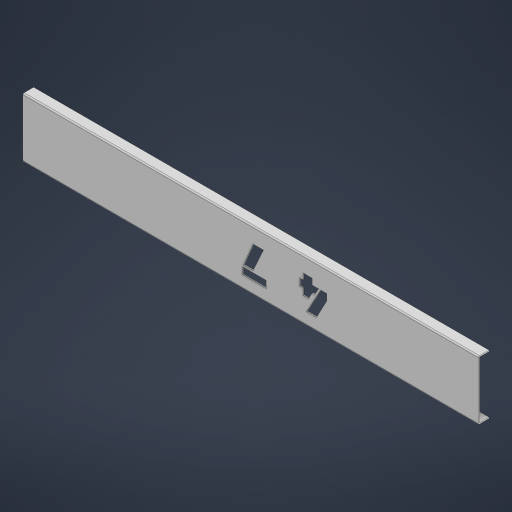
# Autodesk Inventor part: Chassis FrontandBack
Saved by Autodesk Inventor 2023 (Build 270158000, 158)
## iProperties
Created: 2022-04-13
Part Number: Chassis FrontandBack
Material: Generic
Document SubType Name: Modeling
Designer: timmy
Density: 1 g/cm^3
Appearance: Default
Author: timmy
Autodesk Inventor part; units mm, degrees
ref_plane "YZ Plane" through (0, 0, 0) normal (1, 0, 0) x (0, 1, 0)
ref_plane "XZ Plane" through (0, 0, 0) normal (0, 1, 0) x (-1, 0, 0)
ref_plane "XY Plane" through (0, 0, 0) normal (0, 0, 1) x (1, 0, 0)
sketch "Sketch1" plane through (0, 0, 0) normal (0, 0, 1) x (1, 0, 0)
  line L0 (0, 0) -> (609.6, 0)
  line L1 (609.6, 0) -> (609.6, 76.2)
  line L2 (609.6, 76.2) -> (0, 76.2)
  line L3 (0, 76.2) -> (0, 0)
  dimension "d0" = 609.6
  dimension "d1" = 76.2
  constraints: 8 end point, 2 parallel, 1 horizontal, 1 perpendicular
  measures "d0" distance of L2.end L1.end
  measures "d1" distance of L1.end L0.end
extrude "Extrusion1" add sketch "Sketch1" along normal blind 1.5875
sketch "Sketch2" plane through (0, 76.2, 0) normal (0, 1, 0) x (1, 0, 0)
  line L0 (609.6, 0) -> (0, 0) projected
  line L1 (0, 0) -> (0, -1.5875) projected
  line L2 (609.6, -1.5875) -> (0, -1.5875) projected
  line L3 (609.6, 0) -> (609.6, -1.5875) projected
  line L4 (609.6, -1.5875) -> (0, -1.5875)
  line L5 (0, -1.5875) -> (0, 12.7)
  line L6 (0, 12.7) -> (609.6, 12.7)
  line L7 (609.6, 12.7) -> (609.6, -1.5875)
  dimension "d39" = 12.7
  constraints: 8 end point, 2 parallel, 1 horizontal, 1 perpendicular
  measures "d39" distance between parallel lines of L6 L0
extrude "Extrusion2" add sketch "Sketch2" along normal blind 1.5875
fillet "Fillet1" radius 1.5875 1 edges at (304.8, 77.7875, 1.5875)
sketch "Sketch3" plane through (0, 0, 0) normal (0, -1, 0) x (1, 0, 0)
  line L0 (609.6, 0) -> (0, 0) projected
  line L1 (0, -12.7) -> (0, 0) projected
  line L2 (609.6, -12.7) -> (0, -12.7) projected
  line L3 (609.6, 0) -> (609.6, -12.7) projected
extrude "Extrusion3" add sketch "Sketch3" along normal blind 1.5875
sketch "Sketch4" plane through (0, 76.2, -12.7) normal (-1, 0, 0) x (0, 0, 1)
  line L0 (12.7, -76.2) -> (0, -76.2) projected
  line L1 (0, -76.2) -> (0, -77.7875) projected
  line L2 (12.7, -77.7875) -> (0, -77.7875) projected
  line L3 (12.7, -76.2) -> (12.7, -77.7875) projected
  arc A0 (14.2875, 0) -> (12.7, 1.5875) centre (12.7, 0) ccw projected
  line L4 (0, 1.5875) -> (12.7, 1.5875) projected
  line L5 (0, 0) -> (0, 1.5875) projected
  line L6 (0, 0) -> (12.7, 0) projected
  line L7 (12.7, 0) -> (12.7, -76.2) projected
  line L8 (12.7, -76.2) -> (14.2875, -76.2) projected
  line L9 (14.2875, -76.2) -> (14.2875, 0) projected
  line L10 (12.7, -76.2) -> (14.2875, -76.2)
  line L11 (14.2875, -76.2) -> (14.2875, -77.7875)
  line L12 (14.2875, -77.7875) -> (12.7, -77.7875)
  line L13 (12.7, -77.7875) -> (12.7, -76.2)
  constraints: 8 end point, 2 parallel, 1 horizontal, 1 perpendicular
extrude "Extrusion4" add sketch "Sketch4" against normal up to surface (609.6 mm away) contours L8 L11 L12 L3
fillet "Fillet2" radius 1.5875 1 edges at (304.8, -1.5875, 1.5875)
sketch "Sketch5" plane through (0, 0, 1.5875) normal (0, 0, 1) x (1, 0, 0)
  line L0 (391.8077, 9.2075) -> (217.7923, 9.2075) construction
  line L1 (217.7923, 9.2075) -> (217.7923, 67.0009) construction
  line L2 (217.7923, 67.0009) -> (391.8077, 67.0009) construction
  line L3 (391.8077, 67.0009) -> (391.8077, 9.2075) construction
  line L4 (392.9131, 14.4793) -> (379.4788, 14.4793)
  line L5 (379.4788, 14.4793) -> (398.5016, 49.12)
  line L6 (398.5016, 49.12) -> (406.8657, 49.12)
  line L7 (406.8657, 49.12) -> (406.8657, 40.7559)
  line L8 (406.8657, 40.7559) -> (392.9131, 14.4793)
  line L9 (390.2115, 39.5716) -> (386.9546, 39.5716)
  line L10 (386.9546, 39.5716) -> (382.3899, 30.9748)
  line L11 (382.3899, 30.9748) -> (374.9266, 30.9748)
  line L12 (374.9266, 30.9748) -> (374.9266, 39.5716)
  line L13 (374.9266, 39.5716) -> (369.7453, 39.5716)
  line L14 (369.7453, 39.5716) -> (369.7453, 49.12)
  line L15 (369.7453, 49.12) -> (374.9266, 49.12)
  line L16 (374.9266, 49.12) -> (374.9266, 57.1881)
  line L17 (374.9266, 57.1881) -> (386.9546, 57.1881)
  line L18 (386.9546, 57.1881) -> (386.9546, 49.12)
  line L19 (386.9546, 49.12) -> (395.8369, 49.12)
  line L20 (395.8369, 49.12) -> (390.2115, 39.5716)
  line L21 (308.0211, 26.3513) -> (322.0801, 57.1881)
  line L22 (322.0801, 57.1881) -> (308.0211, 57.1881)
  line L23 (308.0211, 57.1881) -> (295.1504, 26.3513)
  line L24 (295.1504, 26.3513) -> (308.0211, 26.3513)
  line L25 (325.5793, 14.4793) -> (325.5793, 23.894)
  line L26 (325.5793, 23.894) -> (293.6633, 23.894)
  line L27 (325.5793, 14.4793) -> (293.6633, 14.4793)
  line L28 (293.6633, 14.4793) -> (293.6633, 23.894)
  line L29 (352.5859, 14.2935) -> (352.5859, 45.4091)
  line L30 (350.864, 47.7439) -> (345.5928, 47.7439)
  line L31 (345.5928, 47.7439) -> (345.5928, 57.5211)
  line L32 (365.0153, 45.4091) -> (365.0153, 26.3513)
  arc A0 (352.5859, 45.4091) -> (350.901, 47.695) centre (350.286, 45.4778) ccw
  arc A1 (352.5859, 14.2935) -> (365.0153, 26.3513) centre (353.0272, 26.2737) ccw
  arc A2 (343.0715, 27.1984) -> (347.3973, 23.4081) centre (346.8949, 27.1984) ccw
  line L33 (343.0715, 57.5844) -> (343.0715, 27.1984)
  line L34 (349.8722, 23.894) -> (349.8722, 14.2935)
  line L35 (349.8722, 14.2935) -> (343.6768, 14.2935)
  arc A3 (330.9215, 25.1088) -> (343.6768, 14.2935) centre (342.4037, 25.7213) ccw
  line L36 (330.9215, 25.1088) -> (330.4406, 46.1275)
  arc A4 (343.0715, 57.5844) -> (330.4406, 46.1275) centre (341.718, 46.3855) ccw
  line L37 (345.5928, 57.5211) -> (352.5859, 57.5211)
  arc A5 (365.0153, 45.4091) -> (352.5859, 57.5211) centre (353.9551, 46.4926) ccw
  line L38 (609.6, 0) -> (609.6, 76.2) projected
  line L39 (0, 0) -> (0, 76.2) projected
  line L40 (609.6, 0) -> (0, 0) projected
  line L41 (0, 76.2) -> (609.6, 76.2) projected
  point P0 (0, 38.1)
  point P1 (217.7923, 38.1042)
  constraints: 68 end point, 12 point on circle, 10 perpendicular, 8 point on line, 7 horizontal, 6 centre point, 5 vertical, 4 parallel, 2 midpoint, 2 tangent, 2 other
extrude "Extrusion8" cut sketch "Sketch5" against normal blind 25.4 contours L4 L5 L6 L7 L8 | L9 L10 L11 L12 L13 L14 L15 L16 L17 L18 L19 L20 | L24 L23 L22 L21 | L27 L28 L26 L25
body "Solid1"
